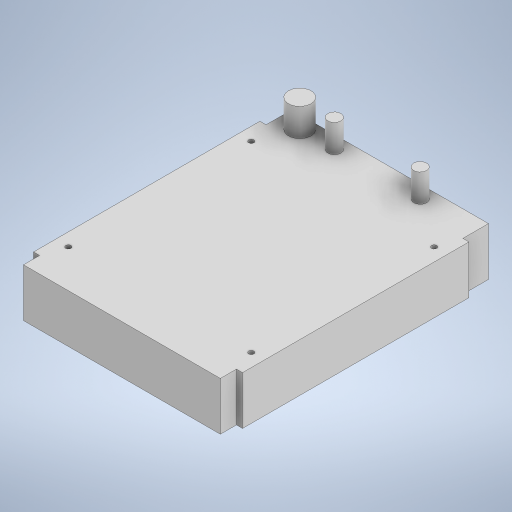
# Autodesk Inventor part: Radiator
Saved by Autodesk Inventor 2023 (Build 270158000, 158)
## iProperties
Created: 2023-08-19
Part Number: Radiator
Material: Generic
Document SubType Name: Modeling
Designer: plebbb
Density: 1 g/cm^3
Appearance: Default
Author: plebbb
Autodesk Inventor part; units mm, degrees
ref_plane "YZ Plane" through (0, 0, 0) normal (1, 0, 0) x (0, 1, 0)
ref_plane "XZ Plane" through (0, 0, 0) normal (0, 1, 0) x (-1, 0, 0)
ref_plane "XY Plane" through (0, 0, 0) normal (0, 0, 1) x (1, 0, 0)
sketch "Sketch1" plane through (0, 0, 0) normal (0, 1, 0) x (-1, 0, 0)
  line L0 (0, 0) -> (120, 0)
  line L1 (120, 0) -> (120, -130)
  line L2 (120, -130) -> (0, -130)
  line L3 (0, -130) -> (0, 0)
  line L4 (112.5, -12.5) -> (7.5, -12.5) construction
  line L5 (7.5, -12.5) -> (7.5, -117.5) construction
  line L6 (7.5, -117.5) -> (112.5, -117.5) construction
  line L7 (112.5, -117.5) -> (112.5, -12.5) construction
  circle A0 centre (112.5, -12.5) radius 1.524
  circle A1 centre (112.5, -117.5) radius 1.524
  circle A2 centre (7.5, -12.5) radius 1.524
  circle A3 centre (7.5, -117.5) radius 1.524
  line L8 (116.5, -130) -> (3.5, -130)
  line L9 (3.5, -130) -> (3.5, -144.7)
  line L10 (3.5, -144.7) -> (116.5, -144.7)
  line L11 (116.5, -144.7) -> (116.5, -130)
  line L12 (116.5, 0) -> (3.5, 0)
  line L13 (3.5, 0) -> (3.5, 9.25)
  line L14 (3.5, 9.25) -> (116.5, 9.25)
  line L15 (116.5, 9.25) -> (116.5, 0)
  point P0 (112.5, -65)
  point P1 (120, -65)
  point P2 (60, -117.5)
  point P3 (60, -130)
  point P4 (60, -144.7)
  point P5 (60, -130)
  point P6 (116.5, 4.625)
  point P7 (116.5, -137.35)
  point P8 (3.5, 0)
  point P9 (3.5, -130)
  dimension "d0" = 130
  dimension "d1" = 120
  dimension "d2" = 105
  dimension "d3" = 3.048
  dimension "d4" = 14.7
  dimension "d5" = 113
  dimension "d6" = 9.25
  constraints: 32 end point, 8 midpoint, 8 parallel, 4 centre point, 4 coincident, 4 horizontal, 4 perpendicular, 4 vertical alignment, 3 equal radius, 2 equal length, 2 point on line, 1 horizontal alignment
  measures "d0" distance of L0.end L1.end
  measures "d1" distance of L1.end L2.end
  measures "d2" distance of L6.end L4.start
  measures "d3" diameter of A0
  measures "d4" distance between parallel lines of L2 L10
  measures "d5" distance of L9.end L10.end
  measures "d6" distance between parallel lines of L0 L14
extrude "Extrusion1" add sketch "Sketch1" along normal blind 27.75
sketch "Sketch2" plane through (0, 27.75, 0) normal (0, 1, 0) x (1, 0, 0)
  circle A0 centre (-104.5, 137.35) radius 6.5
  circle A1 centre (-84.65, 137.35) radius 3.75
  circle A2 centre (-35.35, 137.35) radius 3.75
  line L0 (-116.5, 144.7) -> (-116.5, 130) projected
  line L1 (-3.5, 130) -> (-3.5, 144.7) projected
  point P0 (0, 0)
  point P1 (-116.5, 137.35)
  point P2 (-116.5, 137.35)
  point P3 (-116.5, 137.35)
  point P4 (-116.5, 137.35)
  point P5 (-3.5, 137.35)
  dimension "d9" = 13
  dimension "d10" = 7.5
  dimension "d11" = 12
  dimension "d12" = 31.85
  dimension "d13" = 31.85
  constraints: 5 midpoint, 3 centre point, 3 horizontal alignment, 1 equal radius
  measures "d9" diameter of A0
  measures "d10" diameter of A1
  measures "d11" distance of A0.centre point (-116.5, 137.35)
  measures "d12" distance of A1.centre point (-116.5, 137.35)
  measures "d13" distance of point (-3.5, 137.35) A2.centre
extrude "Extrusion2" add sketch "Sketch2" along normal blind 16
equation "\"d13\" = d12"
body "Solid1"
